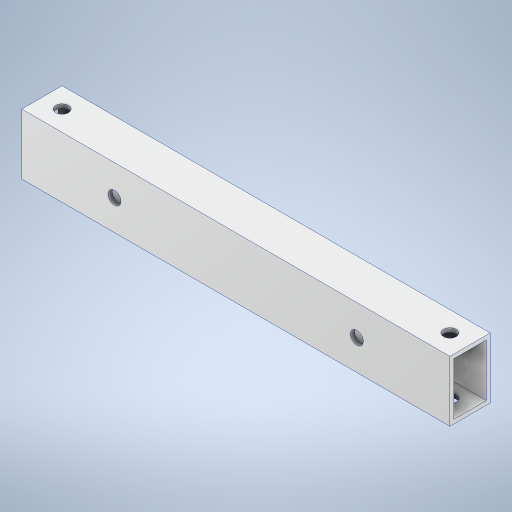
# Autodesk Inventor part: link2_pipe1
Saved by Autodesk Inventor 2024 (Build 280153000, 153)
## iProperties
Created: 2024-12-13
Part Number: link2_pipe1
Material: アルミニウム 6061
Document SubType Name: Modeling
Designer: hirek
Density: 2.7 g/cm^3
Appearance: アルミニウム - フラット
Author: hirek
Autodesk Inventor part; units mm, degrees
ref_plane "YZ Plane" through (0, 0, 0) normal (1, 0, 0) x (0, 1, 0)
ref_plane "XZ Plane" through (0, 0, 0) normal (0, 1, 0) x (-1, 0, 0)
ref_plane "XY Plane" through (0, 0, 0) normal (0, 0, 1) x (1, 0, 0)
sketch "スケッチ1" plane through (0, 0, 0) normal (1, 0, 0) x (0, 1, 0)
  line L0 (0, 0) -> (15, 0)
  line L1 (15, 0) -> (15, -10)
  line L2 (15, -10) -> (0, -10)
  line L3 (0, -10) -> (0, 0)
  line L4 (1, -1) -> (14, -1)
  line L5 (14, -1) -> (14, -9)
  line L6 (14, -9) -> (1, -9)
  line L7 (1, -9) -> (1, -1)
  dimension "d0" = 15
  dimension "d1" = 10
  dimension "d2" = 13
  dimension "d3" = 8
  dimension "d4" = 1
  dimension "d5" = 1
  constraints: 16 end point, 4 parallel, 2 horizontal, 2 perpendicular
  measures "d0" distance of L1.end L2.end
  measures "d1" distance of L0.end L1.end
  measures "d2" distance of L5.end L6.end
  measures "d3" distance of L4.end L5.end
  measures "d4" distance between parallel lines of L5 L1
  measures "d5" distance between parallel lines of L2 L6
extrude "押し出し1" add sketch "スケッチ1" along normal blind 106
sketch "スケッチ2" plane through (0, 15, 0) normal (0, 1, 0) x (1, 0, 0)
  line L0 (0, 9) -> (0, 1) projected
  line L1 (0, 5) -> (120, 5)
  line L2 (106, 10) -> (106, 0) projected
  point P0 (0, 0)
  point P1 (5, 5)
  point P2 (101, 5)
  point P3 (106, 0)
  dimension "d8" = 5
  dimension "d9" = 5
  constraints: 2 end point, 2 point on line, 1 horizontal, 1 midpoint, 1 other
  measures "d8" distance from line of point (5, 5) L0
hole "穴1" at (5, 15, -5) at (101, 15, -5) direction (0, -1, 0) diameter 3.2 end through all
sketch "スケッチ3" plane through (0, 0, 0) normal (0, 0, 1) x (1, 0, 0)
  line L0 (0, 0) -> (0, 15) projected
  line L1 (0, 7.5) -> (106, 7.5)
  line L2 (106, 0) -> (106, 15) projected
  point P0 (23, 7.5)
  point P1 (83, 7.5)
  point P2 (53, 7.5)
  dimension "d17" = 30
  dimension "d18" = 30
  constraints: 3 midpoint, 2 end point, 2 point on line
  measures "d17" distance of point (23, 7.5) point (53, 7.5)
  measures "d18" distance of point (83, 7.5) point (53, 7.5)
hole "穴2" at (23, 7.5, 0) at (83, 7.5, 0) direction (0, 0, -1) diameter 3.2 end through all
